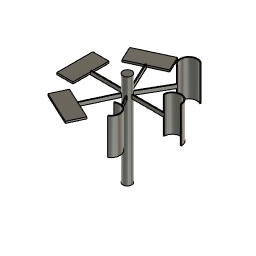
Wind turbine v1 (Autodesk Fusion 360 design; units mm, degrees)
Autodesk Fusion 360 part; units mm, degrees
note: some values were not read from the file. Chosen so that the rebuilt part matches the saved one: which face or edge a step refers to. Set by a fixed rule: which sketch regions a step uses.
sketch "Sketch1" plane through (0, 0, 0) normal (0, 0, 1) x (1, 0, 0)
  arc A0 (50, 0) -> (-50, 0) centre (0, 0) ccw
  arc A1 (45, 0) -> (-45, 0) centre (0, 0) ccw
  line L0 (-50, 0) -> (-45, 0)
  line L1 (45, 0) -> (50, 0)
  dimension "d1" = 100
  dimension "d2" = 90
  dimension "d3" = 100
  constraint coincident A0.centre A1.centre
  constraint horizontal L0
  constraint coincident A1.start L0
  constraint collinear L0 L1
  measures "d1" diameter of A0
  measures "d2" diameter of A1
  measures "d3" distance of A0.end A0.start
extrude "Extrude1" add sketch "Sketch1" along normal mid plane 200 makes body 1
sketch "Sketch2" plane through (0, 0, 0) normal (0, 0, 1) x (1, 0, 0)
  line L0 (-50, 0) -> (-250, 0)
  line L1 (-50, 5) -> (-250, 5)
  line L2 (-250, 5) -> (-250, 0)
  line L3 (-50, 5) -> (-49, 5)
  line L4 (-49, 5) -> (-50, 0)
  dimension "d6" = 200
  constraint horizontal L0
  constraint parallel L0 L1
  constraint perpendicular L0 L2
  constraint parallel L1 L3
  measures "d6" distance of L0.start L0.end
extrude "Extrude2" add sketch "Sketch2" along normal mid plane 20 bodies 1
sketch "Sketch3" plane through (-250, 0, 0) normal (-1, 0, 0) x (0, -1, 0)
  line L0 (0, -10) -> (0, 10)
  line L1 (0, 10) -> (-5, 10)
  line L2 (-5, 10) -> (-5, -10)
  line L3 (-5, -10) -> (0, -10)
sketch "Sketch4" plane through (-250, 0, 0) normal (-1, 0, 0) x (0, -1, 0)
sketch "Sketch5" plane through (0, 0, 0) normal (0, 0, 1) x (1, 0, 0)
  circle A0 centre (-250, 0) radius 25
  dimension "d9" = 50
  measures "d9" diameter of A0
extrude "Extrude3" add sketch "Sketch5" along normal blind 100 and the other way blind 425 bodies 1
pattern_circular "C-Pattern1" count 3 over 120 about axis through (-250, 0, -1112.5) along (0, 0, -1) both ways of bodies 1 makes body 2 at (-159.3173, 180.1426, -3.3333) makes body 3 at (-139.3332, -168.6048, -3.3333)
sketch "Sketch6" plane through (0, 0, 0) normal (0, 0, 1) x (1, 0, 0)
  line L0 (-270, 0) -> (-455, 0)
  line L1 (-270, 0) -> (-270, 5)
  line L2 (-270, 5) -> (-455, 5)
  line L3 (-455, 5) -> (-455, 0)
  dimension "d16" = 185
  constraint horizontal L0
  constraint perpendicular L0 L1
  constraint perpendicular L1 L2
  constraint perpendicular L0 L3
  measures "d16" distance of L0.start L0.end
extrude "Extrude4" add sketch "Sketch6" along normal mid plane 20 bodies 1 2 3
sketch "Sketch7" plane through (-455, 0, 0) normal (-1, 0, 0) x (0, -1, 0)
  line L0 (0, -10) -> (0, 10)
  line L1 (0, 10) -> (-5, 10)
  line L2 (-5, 10) -> (-5, -10)
  line L3 (-5, -10) -> (0, -10)
  line L4 (97.4991, 5.0038) -> (-102.5009, 5.0038)
  line L5 (-102.5009, 5.0038) -> (-102.5009, -4.9962)
  line L6 (-102.5009, -4.9962) -> (97.4991, -4.9962)
  line L7 (97.4991, -4.9962) -> (97.4991, 5.0038)
  line L8 (97.4991, 5.0038) -> (-102.5009, -4.9962) construction
  line L9 (-102.5009, 5.0038) -> (97.4991, -4.9962) construction
  point P0 (-2.5009, 0.0038)
  dimension "d19" = 200
  dimension "d20" = 10
  constraint horizontal L4
  constraint perpendicular L4 L5
  constraint parallel L4 L6
  constraint parallel L5 L7
  constraint coincident L8 P0
  constraint coincident L9 P0
  measures "d19" distance of L5.end L6.end
  measures "d20" distance of L4.end L5.end
extrude "Extrude5" add sketch "Sketch7" along normal blind 90 contours L0 L2 L4 L6 | L0 L4 L6 L7 | L2 L4 L5 L6 bodies 1
pattern_circular "C-Pattern2" count 3 over 130 about axis through (-250, 0, -1112.5) along (0, 0, 1) both ways of "Extrude4", "Extrude5"
